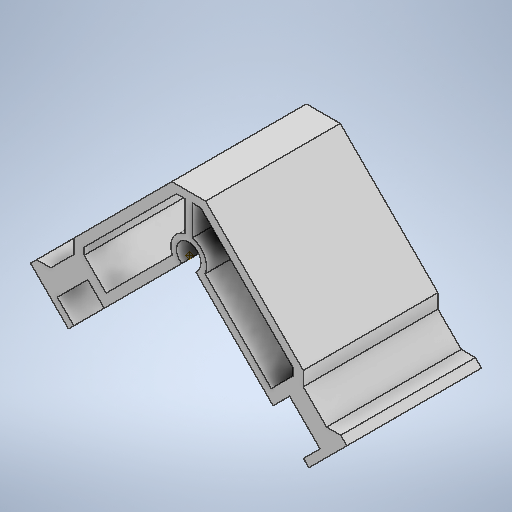
# Autodesk Inventor part: BRA-12 ESCUADRA UNIÓN 45 10 mm
Saved by Autodesk Inventor 2025 (Build 290162000, 162)
## iProperties
Created: 2026-02-04
Part Number: BRA-12 ESCUADRA UNIÓN 45 10 mm
Material: Generic
Document SubType Name: Modeling
Designer: Frank
Density: 1 g/cm^3
Appearance: Default
Author: Frank
Autodesk Inventor part; units mm, degrees
ref_plane "YZ Plane" through (0, 0, 0) normal (1, 0, 0) x (0, 1, 0)
ref_plane "XZ Plane" through (0, 0, 0) normal (0, 1, 0) x (-1, 0, 0)
ref_plane "XY Plane" through (0, 0, 0) normal (0, 0, 1) x (1, 0, 0)
sketch "Sketch1" plane through (0, 0, 0) normal (0, 0, 1) x (1, 0, 0)
  line L0 (-0.7, 9.467) -> (-2.4, 9.467)
  line L1 (-2.4, 9.467) -> (-20.6434, -8.7764)
  line L2 (-20.6434, -8.7764) -> (-20.6434, -10.1764)
  line L3 (-20.6434, -10.1764) -> (-16.3229, -14.4968)
  line L4 (-16.3229, -14.4968) -> (-3.2414, -1.4153)
  line L5 (-22.6434, -8.2308) -> (-3.3393, 11.0732)
  line L6 (-22.6434, -8.2308) -> (-22.6434, -11.0308)
  line L7 (-27.2408, -15.6282) -> (-22.6434, -11.0308)
  line L8 (-30.0408, -15.6282) -> (-31.2428, -16.8303)
  line L9 (-31.2428, -16.8303) -> (-23.7475, -24.3256)
  line L10 (-16.6765, -17.2545) -> (-19.9434, -13.9876)
  line L11 (-19.9434, -13.9876) -> (-25.9538, -19.998)
  line L12 (-25.9538, -19.998) -> (-22.6869, -23.2649)
  line L13 (-23.7475, -24.3256) -> (-22.6869, -23.2649)
  line L14 (-16.6765, -17.2545) -> (-1.4029, -1.981)
  line L15 (-30.0408, -15.6282) -> (-27.2408, -15.6282)
  line L16 (3.3393, 11.0732) -> (-3.3393, 11.0732)
  line L17 (-0.7, 3.467) -> (-0.7, 9.467)
  line L18 (0, 12.3968) -> (0, -27.803) construction
  line L19 (0.7, 9.467) -> (2.4, 9.467)
  line L20 (2.4, 9.467) -> (20.6434, -8.7764)
  line L21 (20.6434, -8.7764) -> (20.6434, -10.1764)
  line L22 (20.6434, -10.1764) -> (16.3229, -14.4968)
  line L23 (16.3229, -14.4968) -> (3.2414, -1.4153)
  line L24 (22.6434, -8.2308) -> (3.3393, 11.0732)
  line L25 (22.6434, -8.2308) -> (22.6434, -11.0308)
  line L26 (27.2408, -15.6282) -> (22.6434, -11.0308)
  line L27 (30.0408, -15.6282) -> (31.2428, -16.8303)
  line L28 (31.2428, -16.8303) -> (23.7475, -24.3256)
  line L29 (16.6765, -17.2545) -> (19.9434, -13.9876)
  line L30 (19.9434, -13.9876) -> (25.9538, -19.998)
  line L31 (25.9538, -19.998) -> (22.6869, -23.2649)
  line L32 (23.7475, -24.3256) -> (22.6869, -23.2649)
  line L33 (16.6765, -17.2545) -> (1.4029, -1.981)
  line L34 (30.0408, -15.6282) -> (27.2408, -15.6282)
  line L35 (0.7, 3.467) -> (0.7, 9.467)
  arc A0 (1.4029, -1.981) -> (-1.4029, -1.981) centre (0, 0) ccw
  arc A1 (3.2414, -1.4153) -> (0.7, 3.467) centre (0, 0) ccw
  arc A2 (-0.7, 3.467) -> (-3.2414, -1.4153) centre (0, 0) ccw
  dimension "d77" = 1.8
  dimension "d83" = 27.3
  dimension "d84" = 135
  dimension "d87" = 2.8
  dimension "d88" = 135
  dimension "d89" = 2.8
  dimension "d90" = 1.7
  dimension "d93" = 4
  dimension "d94" = 1.5
  dimension "d96" = 8.5
  dimension "d100" = 1.4
  dimension "d101" = 2.2
  dimension "d102" = 2
  dimension "d103" = 1.7
  dimension "d104" = 10.6
  dimension "d106" = 135
  dimension "d107" = 25.8
  dimension "d108" = 18.5
  dimension "d109" = 21.6
  dimension "d110" = 6
  dimension "d111" = 0.7
  dimension "d112" = 1.7
  constraints: 72 end point, 19 symmetric about line, 7 parallel, 6 point on circle, 4 perpendicular, 3 centre point, 3 vertical, 2 coincident, 1 collinear, 1 horizontal, 1 point on line
  measures "d77" distance between parallel lines of L5 L1
  measures "d83" distance of L5.start L5.end
  measures "d84" angle of L7 L6
  measures "d87" distance of L5.start L6.end
  measures "d88" angle of L15 L7
  measures "d89" distance of L8.start L7.start
  measures "d90" distance of L8.start L8.end
  measures "d93" distance between parallel lines of L11 L7
  measures "d94" distance between parallel lines of L9 L12
  measures "d96" distance between parallel lines of L10 L12
  measures "d100" distance of L1.end L2.end
  measures "d101" distance between parallel lines of L3 L10
  measures "d102" distance between parallel lines of L2 L6
  measures "d103" distance between parallel lines of L4 L14
  measures "d104" distance of L8.end L9.end
  measures "d106" angle of L1 L0
  measures "d107" distance of L0.end L1.end
  measures "d108" distance of L4.end L3.end
  measures "d109" distance of L14.end L10.start
  measures "d110" distance of L17.start L0.start
  measures "d111" distance between parallel lines of L17 L18
  measures "d112" distance of L0.start L0.end
extrude "Extrusion1" add sketch "Sketch1" against normal blind 26.6
body "Solid1"
